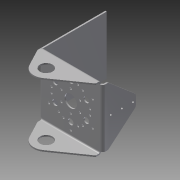
# Autodesk Inventor part: Plate 2 (Back)
Saved by Autodesk Inventor 2014 (Build 180170000, 170)
## iProperties
Created: 2014-01-12
Part Number: Plate 2 (Back)
Material: Steel
Document SubType Name: Sheet Metal
Designer: Andrew Toennies
Density: 7.85 g/cm^3
Sheet Metal Rule: Default
Appearance: Steel
Mass: 1598.73 g
Surface Area: 1395.71 cm^2
Volume: 203.66 cm^3
Author: Andrew Toennies
Autodesk Inventor part; units mm, degrees
ref_plane "YZ Plane" through (0, 0, 0) normal (1, 0, 0) x (0, 1, 0)
ref_plane "XZ Plane" through (0, 0, 0) normal (0, 1, 0) x (-1, 0, 0)
ref_plane "XY Plane" through (0, 0, 0) normal (0, 0, 1) x (1, 0, 0)
sketch "Sketch1" plane through (0, 0, 0) normal (0, 0, 1) x (1, 0, 0)
  circle A0 centre (0, 0) radius 66.675 construction
  circle A1 centre (0, 0) radius 14.2875
  circle A2 centre (0, 41.275) radius 6.3881
  line L0 (0, 0) -> (0, 41.275) construction
  circle A3 centre (0, 41.275) radius 16.637 construction
  circle A4 centre (0, 57.912) radius 2.3812
  circle A5 centre (16.637, 41.275) radius 2.3812
  circle A6 centre (0, 24.638) radius 2.3812
  circle A7 centre (-16.637, 41.275) radius 2.3813
  line L1 (0, 41.275) -> (0, 57.912) construction
  line L2 (-16.637, 41.275) -> (16.637, 41.275) construction
  circle A8 centre (-50.1533, 28.956) radius 2.3812
  circle A9 centre (-44.0637, 6.2294) radius 2.3813
  circle A10 centre (-35.7452, 20.6375) radius 6.3881
  circle A11 centre (-27.4267, 35.0456) radius 2.3812
  circle A12 centre (-21.3371, 12.319) radius 2.3812
  circle A13 centre (-50.1533, -28.956) radius 2.3812
  circle A14 centre (-27.4267, -35.0456) radius 2.3813
  circle A15 centre (-35.7452, -20.6375) radius 6.3881
  circle A16 centre (-44.0637, -6.2294) radius 2.3812
  circle A17 centre (-21.3371, -12.319) radius 2.3812
  circle A18 centre (0, -57.912) radius 2.3812
  circle A19 centre (16.637, -41.275) radius 2.3813
  circle A20 centre (0, -41.275) radius 6.3881
  circle A21 centre (-16.637, -41.275) radius 2.3812
  circle A22 centre (0, -24.638) radius 2.3812
  circle A23 centre (50.1533, -28.956) radius 2.3812
  circle A24 centre (44.0637, -6.2294) radius 2.3813
  circle A25 centre (35.7452, -20.6375) radius 6.3881
  circle A26 centre (27.4267, -35.0456) radius 2.3812
  circle A27 centre (21.3371, -12.319) radius 2.3812
  circle A28 centre (50.1533, 28.956) radius 2.3812
  circle A29 centre (27.4267, 35.0456) radius 2.3813
  circle A30 centre (35.7452, 20.6375) radius 6.3881
  circle A31 centre (44.0637, 6.2294) radius 2.3812
  circle A32 centre (21.3371, 12.319) radius 2.3812
  line L3 (-66.675, 66.675) -> (66.675, 66.675)
  line L4 (66.675, 66.675) -> (66.675, -66.675)
  line L5 (66.675, -66.675) -> (-66.675, -66.675)
  line L6 (-66.675, -66.675) -> (-66.675, 66.675)
  dimension "d2" = 133.35
  dimension "d3" = 28.575
  dimension "d4" = 12.7762
  dimension "d5" = 41.275
  dimension "d6" = 33.274
  dimension "d7" = 4.7625
  dimension "d8" = 4.7625
  dimension "d9" = 4.7625
  dimension "d10" = 4.7625
  dimension "d11" = 360
  measures "d2" diameter of A0
  measures "d3" diameter of A1
  measures "d4" diameter of A2
  measures "d5" distance of L0.start L0.end
  measures "d6" diameter of A3
  measures "d7" diameter of A4
  measures "d8" diameter of A5
  measures "d9" diameter of A6
  measures "d10" diameter of A7
extrude "Plate1" add sketch "Sketch1" along normal blind 3.175
sketch "Sketch3" plane through (66.675, -69.85, 6.35) normal (0, -1, 0) x (1, 0, 0)
  line L0 (-133.35, 0) -> (0, 0)
  line L1 (0, 0) -> (0, 69.85)
  line L2 (0, 69.85) -> (-133.35, 69.85)
  line L3 (-133.35, 69.85) -> (-133.35, 0)
  constraints: 6 end point, 1 horizontal, 1 perpendicular, 1 vertical
edge flange "Flange2" height 76.2 angle 90 thickness 3.175 bend radius 3.175 thickness toward (0, -1, 0) relief straight relief width 3.175 relief depth 1.5875 corner gap 3.175 corner form 0 edges at (0, -66.675, 3.175) (0, 66.675, 3.175) wall of the first edge with corners at (-66.675, -69.85, 6.35) (66.675, -69.85, 6.35) (66.675, -69.85, 76.2) (-66.675, -69.85, 76.2)
bend "Bend2"
corner "Corner2"
sketch "Sketch5" plane through (-66.675, 69.85, 76.2) normal (0, -1, 0) x (1, 0, 0)
  line L0 (38.7453, -36.6683) -> (41.7281, -43.3665) projected
  line L1 (41.7281, -43.3665) -> (49.0204, -44.1324) projected
  line L2 (49.0204, -44.1324) -> (53.3297, -38.2) projected
  line L3 (53.3297, -38.2) -> (50.3469, -31.5018) projected
  line L4 (50.3469, -31.5018) -> (43.0546, -30.736) projected
  line L5 (43.0546, -30.736) -> (38.7453, -36.6683) projected
  line L6 (53.3297, -38.2) -> (38.7453, -36.6683) construction
  line L7 (49.0204, -44.1324) -> (43.0546, -30.736) construction
  circle A0 centre (46.0375, -37.4342) radius 14.2875
  point P0 (66.675, -76.2)
  dimension "d39" = 28.575
  constraints: 4 end point, 2 midpoint, 2 parallel, 1 centre point
  measures "d39" diameter of A0
extrude "Cut2" cut sketch "Sketch5" against normal mid plane 2540 contours L5 L4 L3 L2 L1 L0 | A0
sketch "Sketch7" plane through (69.85, -66.675, -3.175) normal (1, 0, 0) x (0, 1, 0)
  line L0 (133.35, 0) -> (0, 0)
  line L1 (0, 0) -> (0, -69.85)
  line L2 (0, -69.85) -> (133.35, -69.85)
  line L3 (133.35, -69.85) -> (133.35, 0)
  constraints: 6 end point, 1 horizontal, 1 perpendicular, 1 vertical
edge flange "Flange3" height 76.2 angle 90 thickness 3.175 bend radius 3.175 thickness toward (1, 0, 0) relief straight relief width 3.175 relief depth 1.5875 edges at (66.675, 0, 0) wall of the first edge with corners at (69.85, 66.675, -3.175) (69.85, -66.675, -3.175) (69.85, -66.675, -73.025) (69.85, 66.675, -73.025)
bend "Bend3"
corner "Corner3"
sketch "Sketch8" plane through (69.85, -66.675, -73.025) normal (-1, 0, 0) x (0, 0, 1)
  line L0 (0, 133.35) -> (69.85, 133.35) projected
  line L1 (0, 133.35) -> (0, 0) projected
  line L2 (0, 0) -> (69.85, 0) projected
  line L3 (0, 79.375) -> (63.5, 133.35)
  line L4 (0, 53.975) -> (63.5, 0)
  point P0 (73.025, 66.675)
  dimension "d58" = 25.4
  dimension "d59" = 53.975
  dimension "d60" = 6.35
  dimension "d61" = 6.35
  constraints: 4 end point, 4 point on line
  measures "d58" distance of L4.start L3.start
  measures "d59" distance from line of L2 L4.start
  measures "d60" distance of L0.end L3.end
  measures "d61" distance of L2.end L4.end
extrude "Cut4" cut sketch "Sketch8" against normal blind 3.175
fillet "Fillet2" radius 6.35 4 edges at (71.4375, -66.675, -9.525) (71.4375, -12.7, -73.025) (71.4375, 12.7, -73.025) (71.4375, 66.675, -9.525)
sketch "Sketch9" plane through (69.85, -66.675, -3.175) normal (-1, 0, 0) x (0, 0, 1)
  arc A0 (-61.4313, 66.7512) -> (-65.5687, 66.7512) centre (-63.5, 66.675) ccw projected
  arc A1 (-36.0313, 66.7512) -> (-40.1687, 66.7512) centre (-38.1, 66.675) ccw projected
  arc A2 (-10.6313, 66.7512) -> (-14.7687, 66.7512) centre (-12.7, 66.675) ccw projected
  circle A3 centre (-63.5, 66.675) radius 2.0828
  circle A4 centre (-38.1, 66.675) radius 2.0828
  circle A5 centre (-12.7, 66.675) radius 2.0828
  point P0 (3.175, 66.675)
  dimension "d65" = 4.1656
  dimension "d66" = 4.1656
  dimension "d67" = 4.1656
  constraints: 3 centre point, 3 coincident
  measures "d65" diameter of A3
  measures "d66" diameter of A4
  measures "d67" diameter of A5
extrude "Cut5" cut sketch "Sketch9" against normal blind 3.175
sketch "Sketch11" plane through (-69.85, 66.675, -3.175) normal (-1, 0, 0) x (0, -1, 0)
  line L0 (133.35, 0) -> (0, 0)
  line L1 (0, 0) -> (0, -152.4)
  line L2 (0, -152.4) -> (133.35, -152.4)
  line L3 (133.35, -152.4) -> (133.35, 0)
  constraints: 6 end point, 1 horizontal, 1 perpendicular, 1 vertical
edge flange "Flange4" height 158.75 angle 90 thickness 3.175 bend radius 3.175 thickness toward (-1, 0, 0) relief straight relief width 3.175 relief depth 1.5875 edges at (-66.675, 0, 0) wall of the first edge with corners at (-69.85, -66.675, -3.175) (-69.85, 66.675, -3.175) (-69.85, 66.675, -155.575) (-69.85, -66.675, -155.575)
bend "Bend4"
corner "Corner4"
sketch "Sketch13" plane through (-73.025, -66.675, -155.575) normal (-1, 0, 0) x (0, 0, 1)
  line L0 (0, 0) -> (0, 133.35) projected
  line L1 (152.4, 0) -> (0, 0) projected
  line L2 (0, 79.375) -> (25.4, 79.375)
  line L3 (25.4, 79.375) -> (25.4, 53.975)
  line L4 (25.4, 53.975) -> (0, 53.975)
  line L5 (0, 53.975) -> (0, 79.375)
  point P0 (155.575, 66.675)
  dimension "d81" = 25.4
  dimension "d82" = 25.4
  dimension "d83" = 53.975
  constraints: 8 end point, 2 parallel, 1 horizontal, 1 perpendicular, 1 point on line
  measures "d81" distance between parallel lines of L5 L3
  measures "d82" distance between parallel lines of L4 L2
  measures "d83" distance between parallel lines of L1 L4
extrude "Cut6" cut sketch "Sketch13" against normal blind 3.175
sketch "Sketch14" plane through (-66.675, -69.85, 76.2) normal (0, 1, 0) x (1, 0, 0)
  line L0 (0, 0) -> (0, 69.85)
  line L1 (133.35, 0) -> (133.35, 69.85)
  line L2 (0, 0) -> (-63.5, 0)
  line L3 (-63.5, 0) -> (-63.5, 69.85)
  line L4 (-63.5, 69.85) -> (0, 69.85)
  point P0 (66.675, 76.2)
  dimension "d86" = 63.5
  measures "d86" distance of L0.start L2.end
sheet face with bend "Face2" sketch "Sketch14" thickness 3.175 toward (0, -1, 0) bend radius 3.175 relief straight relief width 3.175 relief depth 1.5875
bend "Bend5"
sketch "Sketch15" plane through (-66.675, 73.025, 76.2) normal (0, 1, 0) x (1, 0, 0)
  line L0 (0, 0) -> (0, 69.85)
  line L1 (133.35, 69.85) -> (133.35, 0)
  line L2 (0, 0) -> (-63.5, 0)
  line L3 (-63.5, 0) -> (-63.5, 69.85)
  line L4 (-63.5, 69.85) -> (0, 69.85)
  point P0 (66.675, 76.2)
  dimension "d92" = 63.5
  dimension "d93" = 69.85
  measures "d92" distance of L0.start L2.end
  measures "d93" distance of L2.end L3.end
sheet face with bend "Face3" sketch "Sketch15" thickness 3.175 toward (0, -1, 0) bend radius 3.175 relief straight relief width 3.175 relief depth 1.5875
bend "Bend6"
fillet "Fillet3" radius 6.35 4 edges at (-71.4375, 66.675, -155.575) (-71.4375, -66.675, -155.575) (-71.4375, -12.7, -155.575) (-71.4375, 12.7, -155.575)
sketch "Sketch17" plane through (-73.025, -66.675, -3.175) normal (-1, 0, 0) x (0, 0, 1)
  line L0 (-127, 79.375) -> (-127, 53.975) projected
  line L1 (-127, 53.975) -> (-146.05, 53.975) projected
  line L2 (-152.4, 6.35) -> (-152.4, 47.625) projected
  line L3 (0, 0) -> (-146.05, 0) projected
  line L4 (0, 0) -> (0, 133.35) projected
  line L5 (-146.05, 133.35) -> (0, 133.35) projected
  line L6 (-152.4, 85.725) -> (-152.4, 127) projected
  line L7 (-121.1124, 25.2112) -> (-104.4626, 60.592)
  line L8 (-104.4626, 72.758) -> (-121.1124, 108.1388)
  line L9 (-105.4055, 120.65) -> (-30.165, 120.65)
  line L10 (-105.4055, 12.7) -> (-30.165, 12.7)
  line L11 (-127, 120.65) -> (-12.7, 66.675) construction
  line L12 (-12.7, 66.675) -> (-101.6, 66.675) construction
  line L13 (-12.7, 66.675) -> (-127, 12.7) construction
  line L14 (-101.6, 66.675) -> (-12.7, 12.7) construction
  line L15 (-12.7, 120.65) -> (-101.6, 66.675) construction
  line L16 (-41.018, 69.85) -> (-78.9056, 69.85)
  line L17 (-41.018, 63.5) -> (-78.9056, 63.5)
  line L18 (-28.5172, 114.761) -> (-61.435, 94.7753)
  line L19 (-74.4471, 86.8751) -> (-99.942, 71.396)
  line L20 (-116.8838, 112.3617) -> (-74.7391, 92.46)
  line L21 (-106.7612, 114.604) -> (-64.4385, 94.6183)
  line L22 (-50.6734, 88.1181) -> (-17.2307, 72.3257)
  line L23 (-17.5228, 114.0075) -> (-50.9654, 93.703)
  line L24 (-63.9775, 85.8028) -> (-80.5533, 75.739)
  line L25 (-17.2307, 61.0243) -> (-56.012, 42.7109)
  line L26 (-64.4385, 38.7317) -> (-106.7612, 18.746)
  line L27 (-80.5533, 57.611) -> (-63.9775, 47.5472)
  line L28 (-56.012, 42.7109) -> (-17.5228, 19.3425)
  line L29 (-39.6623, 57.454) -> (-60.974, 47.3901)
  line L30 (-74.7391, 40.89) -> (-116.8838, 20.9883)
  line L31 (-99.942, 61.954) -> (-74.4471, 46.4749)
  line L32 (-61.435, 38.5747) -> (-28.5172, 18.589)
  line L33 (-60.974, 85.9599) -> (-39.6623, 75.896)
  line L34 (-12.7, 111.2936) -> (-12.7, 75.1967)
  line L35 (-12.7, 58.1533) -> (-12.7, 22.0564)
  arc A0 (-116.8838, 112.3617) -> (-121.1124, 108.1388) centre (-118.2396, 109.4907) ccw
  arc A1 (-105.4055, 120.65) -> (-106.7612, 114.604) centre (-105.4055, 117.475) ccw
  arc A2 (-28.5172, 114.761) -> (-30.165, 120.65) centre (-30.165, 117.475) ccw
  arc A3 (-74.4471, 86.8751) -> (-74.7391, 92.46) centre (-76.0948, 89.589) ccw
  arc A4 (-104.4626, 72.758) -> (-99.942, 71.396) centre (-101.5898, 74.1099) ccw
  arc A5 (-80.5533, 75.739) -> (-78.9056, 69.85) centre (-78.9056, 73.025) ccw
  arc A6 (-60.974, 85.9599) -> (-63.9775, 85.8028) centre (-62.3298, 83.0889) ccw
  arc A7 (-41.018, 69.85) -> (-39.6623, 75.896) centre (-41.018, 73.025) ccw
  arc A8 (-78.9056, 63.5) -> (-80.5533, 57.611) centre (-78.9056, 60.325) ccw
  arc A9 (-63.9775, 47.5472) -> (-60.974, 47.3901) centre (-62.3298, 50.2611) ccw
  arc A10 (-39.6623, 57.454) -> (-41.018, 63.5) centre (-41.018, 60.325) ccw
  arc A11 (-12.7, 111.2936) -> (-17.5228, 114.0075) centre (-15.875, 111.2936) ccw
  arc A12 (-50.9654, 93.703) -> (-50.6734, 88.1181) centre (-49.3177, 90.9891) ccw
  arc A13 (-17.2307, 72.3257) -> (-12.7, 75.1967) centre (-15.875, 75.1967) ccw
  arc A14 (-64.4385, 94.6183) -> (-61.435, 94.7753) centre (-63.0827, 97.4892) ccw
  arc A15 (-12.7, 58.1533) -> (-17.2307, 61.0243) centre (-15.875, 58.1533) ccw
  arc A16 (-17.5228, 19.3425) -> (-12.7, 22.0564) centre (-15.875, 22.0564) ccw
  arc A17 (-30.165, 12.7) -> (-28.5172, 18.589) centre (-30.165, 15.875) ccw
  arc A18 (-61.435, 38.5747) -> (-64.4385, 38.7317) centre (-63.0827, 35.8608) ccw
  arc A19 (-106.7612, 18.746) -> (-105.4055, 12.7) centre (-105.4055, 15.875) ccw
  arc A20 (-121.1124, 25.2112) -> (-116.8838, 20.9883) centre (-118.2396, 23.8593) ccw
  arc A21 (-74.7391, 40.89) -> (-74.4471, 46.4749) centre (-76.0948, 43.761) ccw
  arc A22 (-99.942, 61.954) -> (-104.4626, 60.592) centre (-101.5898, 59.2401) ccw
  point P0 (3.175, 66.675)
  dimension "d101" = 12.7
  dimension "d102" = 25.4
  dimension "d103" = 12.7
  dimension "d104" = 12.7
  dimension "d106" = 25.4
  dimension "d107" = 25.4
  dimension "d112" = 3.175
  dimension "d113" = 3.175
  dimension "d118" = 3.175
  dimension "d119" = 3.175
  dimension "d120" = 3.175
  dimension "d121" = 3.175
  dimension "d122" = 3.175
  dimension "d123" = 3.175
  dimension "d124" = 3.175
  dimension "d125" = 3.175
  dimension "d127" = 12.7
  dimension "d128" = 3.175
  constraints: 58 end point, 46 point on circle, 46 tangent, 23 centre point, 22 equal radius, 18 parallel, 11 point on line, 9 collinear, 4 perpendicular, 1 horizontal
  measures "d101" distance from line of L1 L12.end
  measures "d102" distance from line of L0 L12.end
  measures "d103" distance between parallel lines of L5 L9
  measures "d104" distance between parallel lines of L3 L10
  measures "d106" distance from line of L2 L13.end
  measures "d107" distance from line of L6 L11.start
  measures "d112" distance between parallel lines of L16 L12
  measures "d113" distance between parallel lines of L17 L12
  measures "d118" distance between parallel lines of L18 L15
  measures "d119" distance between parallel lines of L20 L11
  measures "d120" distance between parallel lines of L21 L11
  measures "d121" distance between parallel lines of L15 L23
  measures "d122" distance between parallel lines of L27 L14
  measures "d123" distance between parallel lines of L31 L14
  measures "d124" distance between parallel lines of L30 L13
  measures "d125" distance between parallel lines of L13 L25
  measures "d127" distance between parallel lines of L4 L34
  measures "d128" radius of A0
extrude "Cut7" cut sketch "Sketch17" against normal blind 3.175
equation "\"d62\" = Thickness"
equation "\"d68\" = Thickness"
equation "\"d84\" = Thickness"
equation "\"d129\" = Thickness"
equation "\"d23\" = BendReliefWidth"
equation "\"d24\" = BendReliefDepth"
equation "\"d25\" = MinimumRemnant"
equation "\"d26\" = BendRadius"
equation "\"d30\" = CornerReliefSize"
equation "\"d31\" = GapSize"
equation "\"d32\" = JacobiRadiusSize"
equation "\"d48\" = BendReliefWidth"
equation "\"d49\" = BendReliefDepth"
equation "\"d50\" = MinimumRemnant"
equation "\"d51\" = BendRadius"
equation "\"d54\" = BendRadius"
equation "\"d55\" = CornerReliefSize"
equation "\"d56\" = GapSize"
equation "\"d57\" = JacobiRadiusSize"
equation "\"d71\" = BendReliefWidth"
equation "\"d72\" = BendReliefDepth"
equation "\"d73\" = MinimumRemnant"
equation "\"d74\" = BendRadius"
equation "\"d77\" = BendRadius"
equation "\"d78\" = CornerReliefSize"
equation "\"d79\" = GapSize"
equation "\"d80\" = JacobiRadiusSize"
equation "\"d87\" = BendRadius"
equation "\"d88\" = BendReliefWidth"
equation "\"d90\" = MinimumRemnant"
equation "\"d89\" = BendReliefDepth"
equation "\"d91\" = BendRadius"
equation "\"d94\" = BendRadius"
equation "\"d95\" = BendReliefWidth"
equation "\"d97\" = MinimumRemnant"
equation "\"d96\" = BendReliefDepth"
equation "\"d98\" = BendRadius"
equation "\"BendRadius\" = Thickness"
equation "\"BendReliefWidth\" = Thickness"
equation "\"BendReliefDepth\" = 0.5 * Thickness"
equation "\"CornerReliefSize\" = 4 * Thickness"
equation "\"MinimumRemnant\" = 2 * Thickness"
equation "\"TransitionRadius\" = BendRadius"
equation "\"JacobiRadiusSize\" = BendRadius"
equation "\"GapSize\" = Thickness"
equation "\"d12\" = BendRadius"
equation "\"Thickness\" = 3.175"
body "Solid1"
